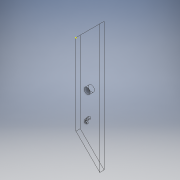
# Autodesk Inventor part: Fata_2
Saved by Autodesk Inventor 2017 (Build 210142000, 142)
## iProperties
Created: 2017-06-02
Part Number: Fata_2
Material: Generic
Document SubType Name: Modeling
Designer: crush
Density: 1 g/cm^3
Appearance: Wood - Painted White
Author: crush
Autodesk Inventor part; units mm, degrees
ref_plane "YZ Plane" through (0, 0, 0) normal (1, 0, 0) x (0, 1, 0)
ref_plane "XZ Plane" through (0, 0, 0) normal (0, 1, 0) x (-1, 0, 0)
ref_plane "XY Plane" through (0, 0, 0) normal (0, 0, 1) x (1, 0, 0)
sketch "Sketch1" plane through (0, 0, 0) normal (0, 1, 0) x (-1, 0, 0)
  line L0 (0, 0) -> (0, -340)
  line L1 (0, 0) -> (-100, 0)
  line L2 (-100, 0) -> (-100, 100)
  line L3 (-100, 100) -> (0, 0)
  line L4 (0, -340) -> (-100, -340)
  line L5 (-100, -340) -> (-100, -440)
  line L6 (-100, -440) -> (0, -340)
  line L7 (-100, -340) -> (-100, 0)
  dimension "d0" = 340
  dimension "d1" = 100
  dimension "d2" = 100
  dimension "d3" = 100
  dimension "d4" = 100
  constraints: 16 end point, 2 horizontal, 2 perpendicular, 2 vertical
  measures "d0" distance of L0.start L0.end
  measures "d1" distance of L0.start L1.end
  measures "d2" distance of L1.end L2.end
  measures "d3" distance of L0.end L4.end
  measures "d4" distance of L4.end L5.end
extrude "Extrusion1" add sketch "Sketch1" along normal blind 18
sketch "Sketch2" plane through (0, 0, 0) normal (0, -1, 0) x (1, 0, 0)
  line L0 (70, -367.7995) -> (70, -407.7995)
  line L1 (25, 17.2005) -> (25, -362.7995)
  arc A0 (51.7994, -181.8328) -> (58.8525, -174.9214) centre (47.1172, -170) ccw
  circle A1 centre (47.1172, -170) radius 12.7255
  line L2 (0, -340) -> (100, -440)
  line L3 (100, 100) -> (0, 0)
  line L4 (100, -440) -> (100, 100)
  line L5 (0, 0) -> (0, -340)
  line L6 (100, 100) -> (100, -440) projected
  line L7 (100, -170) -> (0, -170)
  point P0 (30, 22.2005)
  constraints: 14 end point, 2 centre point, 2 midpoint, 2 point on circle, 1 coincident, 1 point on line
extrude "Extrusion2" cut sketch "Sketch2" against normal blind 20 contours A1 L7 A0 | A1 L7
sketch "Sketch4" plane through (0, 18, 0) normal (0, 1, 0) x (1, 0, 0)
  circle A0 centre (40.0978, 279.5843) radius 3.2826
  line L0 (35.3115, 284.709) -> (45.7543, 284.709)
  line L1 (45.7543, 284.709) -> (45.7543, 291.8643)
  line L2 (45.7543, 291.8643) -> (35.3115, 291.8643)
  line L3 (35.3115, 291.8643) -> (35.3115, 284.709)
  line L4 (0, 340) -> (0, 0)
  line L5 (0, 340) -> (100, 440)
  line L6 (100, -100) -> (100, 440)
  line L7 (100, -100) -> (0, 0)
  dimension "d24" = 6.5652
  constraints: 16 end point, 2 parallel, 1 centre point, 1 horizontal, 1 perpendicular
  measures "d24" diameter of A0
extrude "Extrusion4" cut sketch "Sketch4" against normal blind 10 contours A0
sketch "Sketch6" plane through (0, 0, 0) normal (0, -1, 0) x (1, 0, 0)
  circle A0 centre (40.0978, -279.5843) radius 3.2826 projected
  circle A1 centre (40.0978, -279.5843) radius 3.2826 projected
  circle A2 centre (40.0978, -279.5843) radius 5
  point P0 (0, 0)
  dimension "d14" = 10
  constraints: 1 centre point, 1 coincident
  measures "d14" diameter of A2
sketch "Sketch7" plane through (0, 18, 0) normal (0, 1, 0) x (1, 0, 0)
  circle A0 centre (40.0978, 279.5843) radius 3.2826
  line L0 (35.3115, 284.709) -> (45.7543, 284.709)
  line L1 (45.7543, 284.709) -> (45.7543, 291.8643)
  line L2 (45.7543, 291.8643) -> (35.3115, 291.8643)
  line L3 (35.3115, 291.8643) -> (35.3115, 284.709)
  line L4 (0, 340) -> (0, 0)
  line L5 (0, 340) -> (100, 440)
  line L6 (100, -100) -> (100, 440)
  line L7 (100, -100) -> (0, 0)
  circle A1 centre (40.0978, 279.5843) radius 5
  dimension "d19" = 10
  constraints: 16 end point, 2 centre point, 2 parallel, 1 coincident, 1 horizontal, 1 perpendicular
  measures "d19" diameter of A1
sketch "Sketch8" plane through (0, 0, 0) normal (0, -1, 0) x (1, 0, 0)
  point P0 (0, 0)
extrude "Extrusion7" cut sketch "Sketch7" against normal blind 10 contours A0 | A1
extrude "Extrusion8" cut sketch "Sketch6" against normal blind 18 contours A0
sketch "Sketch9" plane through (0, 0, 0) normal (0, -1, 0) x (1, 0, 0)
  circle A0 centre (40.0978, -279.5843) radius 3.2826 projected
  circle A1 centre (47.1172, -170) radius 12.7255 projected
  line L0 (0, 0) -> (100, 100) projected
  line L1 (0, -340) -> (0, 0) projected
  line L2 (100, -440) -> (0, -340) projected
  line L3 (100, 100) -> (100, -440) projected
  line L4 (35.3092, -291.8611) -> (45.7546, -291.8611)
  line L5 (45.7546, -291.8611) -> (45.7546, -284.7095)
  line L6 (45.7546, -284.7095) -> (35.3092, -284.7095)
  line L7 (35.3092, -284.7095) -> (35.3092, -291.8611)
  constraints: 8 end point, 2 parallel, 1 horizontal, 1 perpendicular
extrude "Extrusion9" cut sketch "Sketch9" against normal blind 5 contours L7 L6 L5 L4
body "Solid1"
